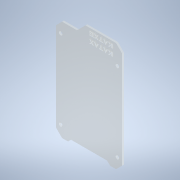
# Autodesk Inventor part: Acrylic Panel
Saved by Autodesk Inventor 2020 (Build 240168000, 168)
## iProperties
Created: 2021-11-22
Part Number: Acrylic Panel
Material: Generic
Document SubType Name: Modeling
Designer: mtkts
Density: 1 g/cm^3
Appearance: Clear
Author: mtkts
Autodesk Inventor part; units mm, degrees
ref_plane "YZ Plane" through (0, 0, 0) normal (1, 0, 0) x (0, 1, 0)
ref_plane "XZ Plane" through (0, 0, 0) normal (0, 1, 0) x (-1, 0, 0)
ref_plane "XY Plane" through (0, 0, 0) normal (0, 0, 1) x (1, 0, 0)
sketch "Sketch1" plane through (0, 0, 0) normal (0, 0, 1) x (1, 0, 0)
  line L0 (5, -135.35) -> (-95.44, -135.35) construction
  line L1 (-95.44, -135.35) -> (-95.44, 3.45) construction
  line L2 (-95.44, 3.45) -> (5, 3.45) construction
  line L3 (5, 3.45) -> (5, -135.35) construction
  line L4 (-100.44, -140.35) -> (10, -140.35)
  line L5 (10, -140.35) -> (10, 8.45)
  line L6 (10, 8.45) -> (-100.44, 8.45)
  line L7 (-100.44, 8.45) -> (-100.44, -140.35)
  circle A0 centre (2.28, -132.2) radius 1.5 projected
  circle A1 centre (-92.72, -132.2) radius 1.5 projected
  circle A2 centre (-92.72, 0.3) radius 1.5 projected
  circle A3 centre (2.28, 0.3) radius 1.5 projected
  circle A4 centre (2.28, -132.2) radius 3
  circle A5 centre (-92.72, -132.2) radius 3
  circle A6 centre (2.28, 0.3) radius 3
  circle A7 centre (-92.72, 0.3) radius 3
  line L8 (-100.44, -140.35) -> (-90.44, -150.35)
  line L9 (-100.44, -140.35) -> (-86.2979, -140.35) construction
  line L10 (-45.22, -140.35) -> (-45.22, -155.35) construction
  line L11 (-90.44, -150.35) -> (10, -150.35) construction
  line L12 (10, -140.35) -> (0, -150.35)
  line L13 (-55.22, -145.35) -> (-35.22, -145.35) construction
  line L14 (-35.22, -145.35) -> (-35.22, -155.35) construction
  line L15 (-35.22, -155.35) -> (-55.22, -155.35)
  line L16 (-55.22, -155.35) -> (-55.22, -145.35) construction
  line L17 (-55.22, -145.35) -> (-35.22, -155.35) construction
  line L18 (-35.22, -145.35) -> (-55.22, -155.35) construction
  line L19 (-55.22, -155.35) -> (-60.22, -150.35)
  line L20 (-35.22, -155.35) -> (-30.22, -150.35)
  line L21 (0, -150.35) -> (-30.22, -150.35)
  line L22 (-60.22, -150.35) -> (-90.44, -150.35)
  line L23 (-96.9045, -136.8145) -> (-88.3689, -145.35) construction
  line L24 (-88.3689, -145.35) -> (-58.1489, -145.35) construction
  line L25 (-58.1489, -145.35) -> (-53.1489, -150.35)
  line L26 (-53.1489, -150.35) -> (-37.2911, -150.35)
  line L27 (-37.2911, -150.35) -> (-32.2911, -145.35)
  line L28 (-32.2911, -145.35) -> (0, -145.35) construction
  line L29 (-32.2911, -145.35) -> (-58.1489, -145.35)
  line L30 (-100.44, 8.45) -> (-90.44, 18.45)
  line L31 (10, 8.45) -> (10, 22.5921)
  line L32 (-90.44, 18.45) -> (-65.44, 18.45)
  line L33 (-65.44, 18.45) -> (-51.2979, 32.5921)
  line L34 (-51.2979, 32.5921) -> (0, 32.5921)
  line L35 (10, 22.5921) -> (0, 32.5921)
  point P0 (0, 0)
  point P1 (-45.22, -150.35)
  point P2 (10, 32.5921)
  dimension "d0" = 5
  dimension "d3" = 6
  dimension "d4" = 6
  dimension "d5" = 6
  dimension "d6" = 6
  dimension "d7" = 14.1421
  dimension "d8" = 45
  dimension "d9" = 15
  dimension "d10" = 45
  dimension "d11" = 20
  dimension "d12" = 10
  dimension "d13" = 45
  dimension "d14" = 45
  dimension "d15" = 5
  dimension "d16" = 45
  dimension "d17" = 10
  dimension "d18" = 25
  dimension "d20" = 135
  dimension "d21" = 14.1421
  dimension "d22" = 10
  dimension "d23" = 10
  constraints: 72 end point, 8 point on line, 7 parallel, 6 horizontal, 4 centre point, 4 coincident, 3 collinear, 3 midpoint, 3 perpendicular, 2 vertical, 1 equal length, 10 other
  measures "d0" distance between parallel lines of L0 L4
  measures "d3" diameter of A4
  measures "d4" diameter of A5
  measures "d5" diameter of A6
  measures "d6" diameter of A7
  measures "d7" distance of L4.start L8.end
  measures "d8" angle of L8 L9
  measures "d9" distance of L10.start L10.end
  measures "d10" angle of L4 L12
  measures "d11" distance of L14.end L15.end
  measures "d12" distance of L13.end L14.end
  measures "d13" angle of L11 L20
  measures "d14" angle of L11 L19
  measures "d15" distance between parallel lines of L15 L26
  measures "d16" angle of L6 L30
  measures "d17" distance from line of L6 L30.end
  measures "d18" distance of L30.end L32.end
  measures "d20" angle of L32 L33
  measures "d21" horizontal distance of L32.end L33.end
  measures "d22" distance of L31.end point (10, 32.592)
  measures "d23" distance of L34.end point (10, 32.592)
extrude "Extrusion1" add sketch "Sketch1" along normal blind 3.175 contours L7 L6 L5 L4 | L4 L12 L21 L20 L15 L19 L22 L8 | L30 L32 L33 L34 L35 L31 L6
sketch "Sketch3" plane through (0, 0, 3.175) normal (0, 0, 1) x (1, 0, 0)
  line L0 (5, 3.45) -> (-95.44, 3.45) construction
  line L1 (9.504, 4.7542) -> (-60.2396, 4.7542) construction
  line L2 (-60.2396, 4.7542) -> (-60.2396, 32.396) construction
  line L3 (-60.2396, 32.396) -> (9.504, 32.396) construction
  line L4 (9.504, 32.396) -> (9.504, 4.7542) construction
  line L5 (-10.7861, 13.0625) -> (-13.4701, 16.4785)
  line L6 (-13.4701, 16.4785) -> (-10.9335, 16.4785)
  line L7 (-10.9335, 16.4785) -> (-8.2495, 13.0625)
  line L8 (-8.2495, 13.0625) -> (-10.9335, 9.6515)
  line L9 (-10.9335, 9.6515) -> (-13.4701, 9.6515)
  line L10 (-13.4701, 9.6515) -> (-10.7861, 13.0625)
  line L11 (-5.8603, 9.6515) -> (-7.8123, 9.6515)
  line L12 (-7.8123, 9.6515) -> (-7.8123, 13.6267)
  line L13 (-7.8123, 13.6267) -> (-7.9343, 13.4691)
  line L14 (-7.9343, 13.4691) -> (-9.2001, 15.0857)
  line L15 (-9.2001, 15.0857) -> (-8.1021, 16.4785)
  line L16 (-8.1021, 16.4785) -> (-5.8603, 16.4785)
  line L17 (-5.8603, 16.4785) -> (-5.8603, 9.6515)
  line L18 (-16.5557, 10.8004) -> (-17.5673, 8.8534)
  line L19 (-17.5673, 8.8534) -> (-21.5171, 16.4785)
  line L20 (-21.5171, 16.4785) -> (-19.4177, 16.4785)
  line L21 (-19.4177, 16.4785) -> (-16.5557, 10.8004)
  line L22 (-17.2776, 13.398) -> (-15.7119, 16.4785)
  line L23 (-15.7119, 16.4785) -> (-13.6125, 16.4785)
  line L24 (-13.6125, 16.4785) -> (-16.2558, 11.3748)
  line L25 (-16.2558, 11.3748) -> (-17.2776, 13.398)
  line L26 (-28.7813, 11.1155) -> (-21.9543, 11.1155)
  line L27 (-21.9543, 11.1155) -> (-20.9783, 9.6515)
  line L28 (-20.9783, 9.6515) -> (-28.7813, 9.6515)
  line L29 (-28.7813, 9.6515) -> (-28.7813, 11.1155)
  line L30 (-24.3943, 11.6035) -> (-26.3413, 11.6035)
  line L31 (-26.3413, 11.6035) -> (-26.3413, 16.4785)
  line L32 (-26.3413, 16.4785) -> (-24.3943, 16.4785)
  line L33 (-24.3943, 16.4785) -> (-24.3943, 11.6035)
  line L34 (-32.1618, 10.8004) -> (-33.1733, 8.8534)
  line L35 (-33.1733, 8.8534) -> (-37.1231, 16.4785)
  line L36 (-37.1231, 16.4785) -> (-35.0237, 16.4785)
  line L37 (-35.0237, 16.4785) -> (-32.1618, 10.8004)
  line L38 (-32.8836, 13.398) -> (-31.3179, 16.4785)
  line L39 (-31.3179, 16.4785) -> (-29.2185, 16.4785)
  line L40 (-29.2185, 16.4785) -> (-31.8618, 11.3748)
  line L41 (-31.8618, 11.3748) -> (-32.8836, 13.398)
  line L42 (-45.1701, 16.4785) -> (-42.6335, 16.4785)
  line L43 (-42.6335, 16.4785) -> (-37.2655, 9.6515)
  line L44 (-37.2655, 9.6515) -> (-39.8021, 9.6515)
  line L45 (-39.8021, 9.6515) -> (-45.1701, 16.4785)
  line L46 (-40.9001, 15.0857) -> (-39.8021, 16.4785)
  line L47 (-39.8021, 16.4785) -> (-37.2655, 16.4785)
  line L48 (-37.2655, 16.4785) -> (-39.6343, 13.4691)
  line L49 (-39.6343, 13.4691) -> (-40.9001, 15.0857)
  line L50 (-41.5355, 11.0444) -> (-42.6335, 9.6515)
  line L51 (-42.6335, 9.6515) -> (-45.1701, 9.6515)
  line L52 (-45.1701, 9.6515) -> (-42.8013, 12.6609)
  line L53 (-42.8013, 12.6609) -> (-41.5355, 11.0444)
  line L54 (-10.7861, 24.8808) -> (-13.4701, 28.2968)
  line L55 (-13.4701, 28.2968) -> (-10.9335, 28.2968)
  line L56 (-10.9335, 28.2968) -> (-8.2495, 24.8808)
  line L57 (-8.2495, 24.8808) -> (-10.9335, 21.4698)
  line L58 (-10.9335, 21.4698) -> (-13.4701, 21.4698)
  line L59 (-13.4701, 21.4698) -> (-10.7861, 24.8808)
  line L60 (-5.8603, 21.4698) -> (-7.8123, 21.4698)
  line L61 (-7.8123, 21.4698) -> (-7.8123, 25.445)
  line L62 (-7.8123, 25.445) -> (-7.9343, 25.2875)
  line L63 (-7.9343, 25.2875) -> (-9.2001, 26.904)
  line L64 (-9.2001, 26.904) -> (-8.1021, 28.2968)
  line L65 (-8.1021, 28.2968) -> (-5.8603, 28.2968)
  line L66 (-5.8603, 28.2968) -> (-5.8603, 21.4698)
  line L67 (-16.5557, 22.6187) -> (-17.5673, 20.6717)
  line L68 (-17.5673, 20.6717) -> (-21.5171, 28.2968)
  line L69 (-21.5171, 28.2968) -> (-19.4177, 28.2968)
  line L70 (-19.4177, 28.2968) -> (-16.5557, 22.6187)
  line L71 (-17.2776, 25.2163) -> (-15.7119, 28.2968)
  line L72 (-15.7119, 28.2968) -> (-13.6125, 28.2968)
  line L73 (-13.6125, 28.2968) -> (-16.2558, 23.1931)
  line L74 (-16.2558, 23.1931) -> (-17.2776, 25.2163)
  line L75 (-28.7813, 22.9338) -> (-21.9543, 22.9338)
  line L76 (-21.9543, 22.9338) -> (-20.9783, 21.4698)
  line L77 (-20.9783, 21.4698) -> (-28.7813, 21.4698)
  line L78 (-28.7813, 21.4698) -> (-28.7813, 22.9338)
  line L79 (-24.3943, 23.4219) -> (-26.3413, 23.4219)
  line L80 (-26.3413, 23.4219) -> (-26.3413, 28.2968)
  line L81 (-26.3413, 28.2968) -> (-24.3943, 28.2968)
  line L82 (-24.3943, 28.2968) -> (-24.3943, 23.4219)
  line L83 (-37.3671, 28.2968) -> (-34.8305, 28.2968)
  line L84 (-34.8305, 28.2968) -> (-29.4625, 21.4698)
  line L85 (-29.4625, 21.4698) -> (-31.9991, 21.4698)
  line L86 (-31.9991, 21.4698) -> (-37.3671, 28.2968)
  line L87 (-33.7325, 22.8627) -> (-34.8305, 21.4698)
  line L88 (-34.8305, 21.4698) -> (-37.3671, 21.4698)
  line L89 (-37.3671, 21.4698) -> (-34.9983, 24.4792)
  line L90 (-34.9983, 24.4792) -> (-33.7325, 22.8627)
  line L91 (-33.0971, 26.904) -> (-31.9991, 28.2968)
  line L92 (-31.9991, 28.2968) -> (-29.4625, 28.2968)
  line L93 (-29.4625, 28.2968) -> (-31.8313, 25.2875)
  line L94 (-31.8313, 25.2875) -> (-33.0971, 26.904)
  line L95 (-38.0483, 23.4219) -> (-40.0003, 23.4219)
  line L96 (-40.0003, 23.4219) -> (-40.0003, 26.8328)
  line L97 (-40.0003, 26.8328) -> (-44.8753, 26.8328)
  line L98 (-44.8753, 26.8328) -> (-44.8753, 28.2968)
  line L99 (-44.8753, 28.2968) -> (-38.0483, 28.2968)
  line L100 (-38.0483, 28.2968) -> (-38.0483, 23.4219)
  line L101 (-44.8753, 22.9338) -> (-38.0483, 22.9338)
  line L102 (-38.0483, 22.9338) -> (-37.0723, 21.4698)
  line L103 (-37.0723, 21.4698) -> (-44.8753, 21.4698)
  line L104 (-44.8753, 21.4698) -> (-44.8753, 22.9338)
  line L105 (-44.8753, 25.8568) -> (-41.9524, 25.8568)
  line L106 (-41.9524, 25.8568) -> (-40.4883, 24.3928)
  line L107 (-40.4883, 24.3928) -> (-44.8753, 24.3928)
  line L108 (-44.8753, 24.3928) -> (-44.8753, 25.8568)
  point P0 (0, 0)
  constraints: 2 other
extrude "Extrusion2" cut sketch "Sketch3" against normal blind 10
sketch "Sketch7" plane through (0, 0, 3.175) normal (0, 0, 1) x (1, 0, 0)
  line L0 (-35.22, -155.35) -> (-25.22, -145.35) projected
  line L1 (-55.22, -155.35) -> (-35.22, -155.35) projected
  line L2 (-65.22, -145.35) -> (-55.22, -155.35) projected
  line L3 (-53.1489, -150.35) -> (-58.1489, -145.35) projected
  line L4 (-37.2911, -150.35) -> (-53.1489, -150.35) projected
  line L5 (-32.2911, -145.35) -> (-37.2911, -150.35) projected
  line L6 (-58.1489, -145.35) -> (-32.2911, -145.35) projected
  line L7 (-32.2911, -145.35) -> (-25.22, -145.35) projected
  line L8 (-65.22, -145.35) -> (-58.1489, -145.35) projected
  line L9 (-65.22, -145.35) -> (-75.44, -145.35) projected
  line L10 (-80.44, -150.35) -> (-75.44, -145.35) projected
  line L11 (-90.44, -150.35) -> (-60.22, -150.35) projected
  line L12 (-15, -145.35) -> (-25.22, -145.35) projected
  line L13 (-15, -145.35) -> (-10, -150.35) projected
  line L14 (-30.22, -150.35) -> (0, -150.35) projected
  line L15 (-1.0355, -147.85) -> (-8.9645, -147.85) projected
  line L16 (-8.9645, -147.85) -> (-11.4645, -145.35) projected
  line L17 (1.4645, -145.35) -> (-11.4645, -145.35) projected
  line L18 (1.4645, -145.35) -> (-1.0355, -147.85) projected
  line L19 (-81.4755, -147.85) -> (-89.4045, -147.85) projected
  line L20 (-78.9755, -145.35) -> (-81.4755, -147.85) projected
  line L21 (-78.9755, -145.35) -> (-91.9045, -145.35) projected
  line L22 (-89.4045, -147.85) -> (-91.9045, -145.35) projected
  point P0 (0, 0)
extrude "Extrusion3" cut sketch "Sketch7" against normal through all contours L1 L2 L8 L3 L4 L5 L7 L0 | L0 L12 L13 L14 | L11 L10 L9 L2 | L15 L16 L17 L18 | L19 L22 L21 L20
equation "\"d5\" = d3"
equation "\"d6\" = d3"
equation "\"d23\" = d22"
body "Solid1"
